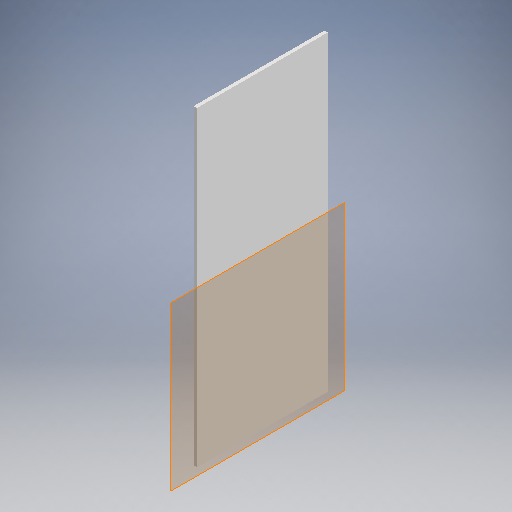
# Autodesk Inventor part: LEFT WALL
Saved by Autodesk Inventor 2025.2 (Build 292293000, 293)
## iProperties
Created: 2025-01-27
Part Number: LEFT WALL
Material: Generic
Document SubType Name: Modeling
Designer: Anna
Density: 1 g/cm^3
Appearance: Default
Author: Anna
Autodesk Inventor part; units mm, degrees
ref_plane "YZ Plane" through (0, 0, 0) normal (1, 0, 0) x (0, 1, 0)
ref_plane "XZ Plane" through (0, 0, 0) normal (0, 1, 0) x (-1, 0, 0)
ref_plane "XY Plane" through (0, 0, 0) normal (0, 0, 1) x (1, 0, 0)
ref_plane "Work Plane1" through (-602.1457, 223.5955, -118.4778) normal (-1, 0, 0) x (0, -1, 0)
sketch "Sketch1" plane through (-602.1457, 223.5955, -118.4778) normal (-1, 0, 0) x (0, -1, 0)
  line L0 (0, 0) -> (0, 1003.3) projected
  line L1 (0, 1003.3) -> (-2387.6, 1003.3)
  line L2 (-2387.6, 1003.3) -> (-2387.6, 0)
  line L3 (-2387.6, 0) -> (0, 0)
  point P0 (223.5955, 118.4778)
  dimension "d0" = 2387.6
  dimension "d1" = 1003.3
  constraints: 6 end point, 2 horizontal
  measures "d0" distance of L0.end L1.end
  measures "d1" distance of L1.end L2.end
extrude "Extrusion1" add sketch "Sketch1" along normal blind 25.4
body "Solid1"
